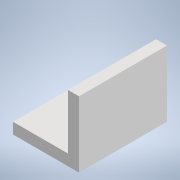
# Autodesk Inventor part: Beschlag_camera
Saved by Autodesk Inventor 2021 (Build 250183000, 183)
## iProperties
Created: 2022-06-27
Part Number: Beschlag_camera
Material: Generisch
Document SubType Name: Modeling
Designer: adria
Mass: 11 g
Surface Area: 53.5 cm^2
Volume: 11 cm^3
Density: 1 g/cm^3
Appearance: Vorgabe
Author: adria
Autodesk Inventor part; units mm, degrees
ref_plane "YZ Plane" through (0, 0, 0) normal (1, 0, 0) x (0, 1, 0)
ref_plane "XZ Plane" through (0, 0, 0) normal (0, 1, 0) x (-1, 0, 0)
ref_plane "XY Plane" through (0, 0, 0) normal (0, 0, 1) x (1, 0, 0)
sketch "Skizze1" plane through (0, 0, 0) normal (0, 0, 1) x (1, 0, 0)
  line L0 (-11.9065, 2.1537) -> (13.0935, 2.1537)
  line L1 (13.0935, 2.1537) -> (13.0935, 27.1537)
  line L2 (13.0935, 27.1537) -> (18.0935, 27.1537)
  line L3 (18.0935, 27.1537) -> (18.0935, -2.8463)
  line L4 (18.0935, -2.8463) -> (-11.9065, -2.8463)
  line L5 (-11.9065, -2.8463) -> (-11.9065, 2.1537)
  point P0 (0, 0)
  dimension "d0" = 5
  dimension "d1" = 5
  dimension "d2" = 30
  dimension "d3" = 30
  constraints: 12 end point, 3 horizontal, 3 vertical
  measures "d0" distance between parallel lines of L4 L0
  measures "d1" distance between parallel lines of L3 L1
  measures "d2" distance between parallel lines of L3 L5
  measures "d3" distance between parallel lines of L2 L4
extrude "Extrusion1" add sketch "Skizze1" along normal blind 40
